dimmer (Autodesk Fusion 360 design; units mm, degrees)
Autodesk Fusion 360 part; units mm, degrees
sketch "Sketch1" plane through (0, 0, 0) normal (0, 1, 0) x (1, 0, 0)
  circle A0 centre (0, 0) radius 1.45
  circle A1 centre (0, 0) radius 15
  dimension "d1" = 2.9
  dimension "d2" = 30
  constraint coincident A0.centre A1.centre
  measures "d1" diameter of A0
  measures "d2" diameter of A1
extrude "Extrude1" add sketch "Sketch1" along normal blind 12
extrude "Extrude2" add sketch "Sketch1" along normal blind 4 contours A0
fillet "Fillet1" radius 1 1 edges at (-1.3519, 12, -0.5243)
sketch "Sketch2" plane through (0, 12, 0) normal (0, 1, 0) x (-1, 0, 0)
  circle A0 centre (0, 0) radius 15
  circle A1 centre (0, 0) radius 2.45
  circle A2 centre (0, 0) radius 7.5
  dimension "d8" = 15
  constraint coincident A0.centre A1.centre
  measures "d8" diameter of A2
extrude "Extrude3" cut sketch "Sketch2" against normal blind 4 contours A0
fillet "Fillet2" radius 3 1 edges at (-13.9849, 0, 5.4242)
fillet "Fillet3" radius 2 1 edges at (-13.9849, 8, -5.4242)
